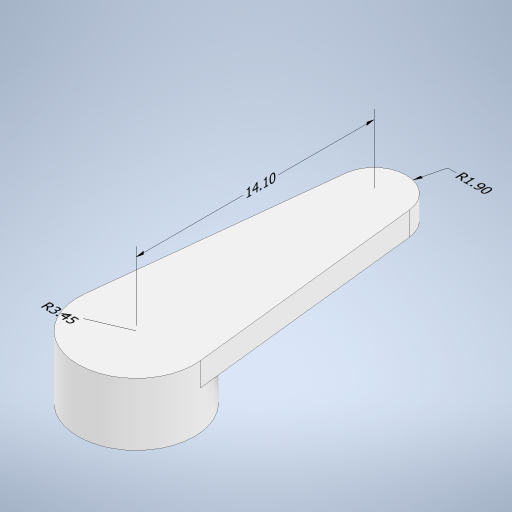
# Autodesk Inventor part: Miusei_hone_short
Saved by Autodesk Inventor 2024.1 (Build 281209000, 209)
## iProperties
Created: 2025-03-02
Part Number: Miusei_hone_short
Material: 一般
Document SubType Name: Modeling
Designer: hibik
Density: 1 g/cm^3
Appearance: 既定
Author: hibik
Autodesk Inventor part; units mm, degrees
ref_plane "YZ Plane" through (0, 0, 0) normal (1, 0, 0) x (0, 1, 0)
ref_plane "XZ Plane" through (0, 0, 0) normal (0, 1, 0) x (-1, 0, 0)
ref_plane "XY Plane" through (0, 0, 0) normal (0, 0, 1) x (1, 0, 0)
sketch "スケッチ1" plane through (0, 0, 0) normal (0, 1, 0) x (-1, 0, 0)
  circle A0 centre (0, 0) radius 3.45
  circle A1 centre (0, 14.1) radius 1.9
  circle A2 centre (0, -14.1) radius 1.9
  line L0 (4.83, 0) -> (-4.83, 0) projected
  line L1 (1.8885, 14.3089) -> (3.4291, 0.3793)
  line L2 (3.4291, -0.3793) -> (1.8885, -14.3089)
  line L3 (-1.8885, -14.3089) -> (-3.4291, -0.3793)
  line L4 (-3.4291, 0.3793) -> (-1.8885, 14.3089)
  dimension "d0" = 6.9
  dimension "d1" = 3.8
  dimension "d3" = 28.2
  constraints: 8 end point, 8 point on circle, 8 tangent, 3 centre point, 2 vertical alignment, 1 coincident, 1 equal radius, 1 symmetric about line
  measures "d0" diameter of A0
  measures "d1" diameter of A1
  measures "d3" distance of A2.centre A1.centre
extrude "押し出し1" add sketch "スケッチ1" along normal blind 1.4 contours L0 A0 | A0 L0 | L2 A2 L3 A0 | A2
sketch "スケッチ2" plane through (0, 0, 0) normal (0, -1, 0) x (1, 0, 0)
  circle A0 centre (0, 0) radius 3.45
  arc A1 (3.4291, -0.3793) -> (-3.4291, -0.3793) centre (0, 0) ccw projected
  point P0 (3.4338, 0.3342)
  constraints: 1 centre point, 1 coincident, 1 concentric
extrude "押し出し2" add sketch "スケッチ2" along normal blind 2.3
